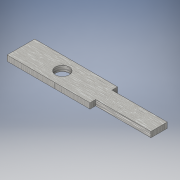
# Autodesk Inventor part: TSV+In
Saved by Autodesk Inventor 2016 (Build 200138000, 138)
## iProperties
Created: 2017-02-28
Part Number: TSV+In
Material: Steel
Document SubType Name: Modeling
Designer: Christer Hoeflinger
Density: 7.85 g/cm^3
Appearance: Polished Brushed
Author: Christer Hoeflinger
Autodesk Inventor part; units mm, degrees
ref_plane "YZ Plane" through (0, 0, 0) normal (1, 0, 0) x (0, 1, 0)
ref_plane "XZ Plane" through (0, 0, 0) normal (0, 1, 0) x (-1, 0, 0)
ref_plane "XY Plane" through (0, 0, 0) normal (0, 0, 1) x (1, 0, 0)
sketch "Sketch1" plane through (0, 0, 0) normal (0, 1, 0) x (-1, 0, 0)
  line L0 (0, 0) -> (76.2, 0)
  line L1 (76.2, 0) -> (76.2, -25.4)
  line L2 (76.2, -25.4) -> (0, -25.4)
  line L3 (0, -25.4) -> (0, 0)
  dimension "d0" = 25.4
  dimension "d1" = 76.2
  constraints: 8 end point, 2 parallel, 1 horizontal, 1 perpendicular
  measures "d0" distance of L2.end L0.start
  measures "d1" distance of L0.start L0.end
extrude "Extrusion1" add sketch "Sketch1" along normal blind 5
sketch "Sketch2" plane through (0, 0, 0) normal (1, 0, 0) x (0, 0, -1)
  line L0 (25.4, 0) -> (0, 0) projected
  line L1 (25.4, 0) -> (25.4, 5) projected
  line L2 (0, 5) -> (25.4, 5) projected
  line L3 (0, 0) -> (0, 5) projected
  line L4 (5.2, 0) -> (20.2, 0)
  line L5 (20.2, 0) -> (20.2, 5)
  line L6 (20.2, 5) -> (5.2, 5)
  line L7 (5.2, 5) -> (5.2, 0)
  dimension "d4" = 15
  dimension "d5" = 25.4
  dimension "d6" = 5.2
  constraints: 8 end point, 2 parallel, 2 point on line, 1 horizontal, 1 perpendicular
  measures "d4" distance between parallel lines of L5 L7
  measures "d5" distance between parallel lines of L1 L3
  measures "d6" distance between parallel lines of L3 L7
extrude "Extrusion2" add sketch "Sketch2" along normal blind 50.8 contours L0 L7 L2 L5
sketch "Sketch4" plane through (0, 5, 0) normal (0, 1, 0) x (1, 0, 0)
  circle A0 centre (-38.1, 12.7) radius 6.35
  line L0 (0, 20.2) -> (0, 25.4) projected
  line L1 (-76.2, 0) -> (0, 0) projected
  dimension "d12" = 12.7
  dimension "d13" = 38.1
  dimension "d14" = 12.7
  constraints: 1 centre point
  measures "d12" diameter of A0
  measures "d13" distance from line of L0 A0.centre
  measures "d14" distance from line of L1 A0.centre
extrude "Extrusion4" cut sketch "Sketch4" against normal blind 50.8
equation "\"d6\" = -0.5 * d4 + 0.5 * d5"
body "Solid1"
